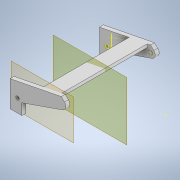
# Autodesk Inventor part: Capping_RotatingArm
Saved by Autodesk Inventor 2022 (Build 260153000, 153)
## iProperties
Created: 2024-05-06
Part Number: Capping_RotatingArm
Material: Generic
Document SubType Name: Modeling
Designer: Gotham City
Density: 1 g/cm^3
Appearance: Default
Author: Gotham City
Autodesk Inventor part; units mm, degrees
ref_plane "YZ Plane" through (0, 0, 0) normal (1, 0, 0) x (0, 1, 0)
ref_plane "XZ Plane" through (0, 0, 0) normal (0, 1, 0) x (-1, 0, 0)
ref_plane "XY Plane" through (0, 0, 0) normal (0, 0, 1) x (1, 0, 0)
sketch "Sketch1" plane through (0, 0, 0) normal (0, 0, 1) x (1, 0, 0)
  line L0 (-13.4159, 40.2876) -> (-44.6613, 29.4467) construction
  circle A0 centre (-45.1029, 22.9379) radius 1.3 projected
  line L1 (-41.8029, 32.9379) -> (-41.8029, 12.9379) projected
  line L2 (-11.7769, 35.5639) -> (-42.4029, 24.9379) construction
  point P0 (0, 0)
sketch "Sketch3" plane through (0, 0, 0) normal (0, 0, 1) x (1, 0, 0)
  line L0 (-41.8029, 32.9379) -> (-41.8029, 12.9379) construction
  line L1 (-41.8029, 12.9379) -> (-50.8029, 12.9379)
  line L2 (-50.8029, 12.9379) -> (-50.8029, 32.9379)
  line L3 (-50.8029, 32.9379) -> (-41.8029, 32.9379)
  line L4 (-41.8029, 32.9379) -> (-41.8029, 12.9379)
  line L5 (-50.8029, 22.9379) -> (-41.8029, 22.9379) construction
  circle A0 centre (-45.1029, 22.9379) radius 1.3 projected
  line L6 (-13.4159, 40.2876) -> (-44.5892, 29.4718)
  line L7 (-44.5892, 29.4718) -> (-41.8029, 21.4414)
  line L8 (-41.8029, 21.4414) -> (-10.6297, 32.2573)
  line L9 (-10.6297, 32.2573) -> (-13.4159, 40.2876)
  line L10 (-13.4159, 40.2876) -> (-41.8029, 21.4414) construction
  line L11 (-44.5892, 29.4718) -> (-10.6297, 32.2573) construction
  line L12 (-42.4029, 24.9379) -> (-11.7769, 35.5639) construction
  line L13 (-13.4159, 40.2876) -> (-44.6613, 29.4467) construction
  circle A1 centre (-11.7769, 35.5639) radius 1.5
  line L14 (-50.8029, 32.9379) -> (-13.4159, 40.2876)
  arc A2 (-10.6297, 32.2573) -> (-9.351, 38.0867) centre (-11.7769, 35.5639) ccw
  line L15 (-11.9413, 40.5775) -> (-9.351, 38.0867)
  line L16 (-13.4159, 40.2876) -> (-11.9413, 40.5775)
  point P0 (0, 0)
  point P1 (-27.6094, 30.8645)
  point P2 (-41.8029, 30.4385)
  point P3 (-11.2853, 34.1468)
  point P4 (-12.2686, 36.981)
  dimension "d0" = 9
  dimension "d1" = 3.5
  dimension "d2" = 0
  dimension "d3" = 3
  dimension "d39" = 125
  constraints: 30 end point, 5 parallel, 4 coincident, 4 midpoint, 4 point on line, 3 point on circle, 2 centre point, 2 perpendicular, 1 collinear, 1 horizontal, 1 tangent
  measures "d0" distance of L2.end L3.end
  measures "d1" distance between parallel lines of L8 L12
  measures "d2" distance between parallel lines of L6 L13
  measures "d3" diameter of A1
  measures "d39" angle of L15 L16
extrude "Extrusion1" add sketch "Sketch3" against normal blind 3 contours L1 L2 L3 L4 L6 L7 | L7 L6 L4 | L4 L6 L9 A1 L8 | L14 L6 L4 L3 | L9 A1 L16 L15 A2
ref_plane "Work Plane2" through (0, 0, 32.5) normal (0, 0, 1) x (1, 0, 0)
ref_plane "Work Plane1" through (0, 0, 65) normal (0, 0, 1) x (1, 0, 0)
sketch "Sketch5" plane through (0, 0, -3) normal (0, 0, -1) x (-1, 0, 0)
  circle A0 centre (11.7769, 35.5639) radius 1.5 projected
  point P0 (0, 0)
  point P1 (11.2853, 34.1468)
  point P2 (12.2686, 36.981)
extrude "Extrusion3" add sketch "Sketch5" against normal blind 1
mirror "Mirror1" about plane through (0, 0, 32.5) normal (0, 0, 1) of "Extrusion1", "Extrusion3"
sketch "Sketch4" plane through (0, 0, 0) normal (0, 0, 1) x (1, 0, 0)
  line L0 (-14.4068, 40.0928) -> (-13.7512, 38.2033)
  line L1 (-13.4159, 40.2876) -> (-44.6613, 29.4467) construction
  line L2 (-13.7512, 38.2033) -> (-26.9777, 33.6143)
  line L3 (-26.9777, 33.6143) -> (-28.2793, 37.3657)
  line L4 (-13.4159, 40.2876) -> (-28.2793, 37.3657)
  line L5 (-50.8029, 32.9379) -> (-11.9413, 40.5775) projected
  circle A0 centre (-11.7769, 35.5639) radius 1.5 construction
  point P0 (0, 0)
  point P1 (-44.6613, 29.4467)
  dimension "d8" = 2
  dimension "d9" = 14
  dimension "d41" = 1
  constraints: 6 end point, 2 point on line, 1 perpendicular, 5 other
  measures "d8" distance of point (-14.407, 40.093) L2.start
  measures "d9" distance of L2.start L2.end
extrude "Extrusion2" add sketch "Sketch4" along normal up to surface (65 mm away)
sketch "Sketch10" plane through (-26.9777, 33.6143, 0) normal (0.3277907, -0.9447504, 0) x (0.9447504, 0.3277907, 0)
  line L0 (14, 0) -> (14, 65) construction
  line L1 (0, 0) -> (0, 65) construction
  circle A0 centre (6, 32.5) radius 5
  line L2 (-45.7867, 32.5) -> (40.0291, 32.5) projected
  point P0 (14.4688, 0)
  dimension "d25" = 10
  dimension "d28" = 8
  constraints: 1 centre point, 1 coincident, 1 point on line
  measures "d25" diameter of A0
  measures "d28" distance from line of A0.centre L0
extrude "Extrusion8" cut sketch "Sketch10" against normal blind 1.1
thicken "Thicken2" operation add thickness 0.1 both sides no extend neighbours yes toward (0.1928936, -0.9812197, 0) faces at (-19.031, 39.1838, 43.3333)
ref_plane "Work Plane3" through (0, 0, 32.5) normal (0, 0, 1) x (1, 0, 0)
equation "\"d4\" = d3"
equation "\"d10\" = d3"
body "Solid1"
